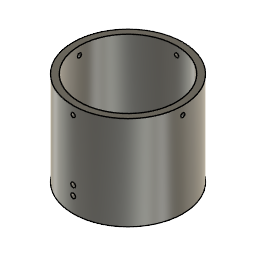
container0306v0.3 (Autodesk Fusion 360 design; units mm, degrees)
Autodesk Fusion 360 part; units mm, degrees
sketch "Sketch1" plane through (0, 0, 0) normal (0, 0, 1) x (1, 0, 0)
  circle A0 centre (0, 0) radius 31.1
  circle A1 centre (0, 0) radius 33.6
  circle A2 centre (0, 0) radius 4
  dimension "d1" = 62.2
  dimension "d2" = 67.2
  dimension "d16" = 8
  constraint coincident A0.centre A1.centre
  constraint concentric A0 A1
  measures "d1" diameter of A0
  measures "d2" diameter of A1
  measures "d16" diameter of A2
extrude "Extrude1" add sketch "Sketch1" along normal blind 60 contours A1
extrude "Extrude2" add sketch "Sketch1" along normal blind 4 contours A0 | A2
ref_plane "WorkPlane1" through (0, -35, 0) normal (0, 1, 0) x (0, 0, 1)
sketch "Sketch2" plane through (0, -35, 0) normal (0, 1, 0) x (1, 0, 0)
  circle A0 centre (0, -10) radius 1.5
  circle A1 centre (0, -16) radius 1.5
  circle A2 centre (0, -54.7) radius 1.3
  line L0 (0, 0) -> (0, -53.4)
  dimension "d25" = 3
  dimension "d26" = 6
  dimension "d27" = 3
  dimension "d32" = 2.6
  constraint coincident L0.start origin
  constraint vertical L0
  constraint coincident A2 L0.end
  measures "d25" diameter of A0
  measures "d26" distance of A0.centre A1.centre
  measures "d27" diameter of A1
  measures "d32" diameter of A2
hole "Hole2" at (0, 0, 0) direction (0, 0, 1) diameter 8 depth 8 tip angle 118
extrude "Extrude4" cut sketch "Sketch2" along normal blind 85 contours A0 L0 | A0 L0 | A1 L0 | A1 L0
extrude "Extrude5" cut sketch "Sketch2" along normal blind 14 contours A2
pattern_circular "C-Pattern2" count 4 over 360 about axis through (0, 0, 1.75) along (0, 0, 1) of 1 faces at (0.3204, -31.9316, 53.4401)
move_face "OffsetFaces1" offset 1.5 1 faces at (5.4983, 33.1471, 25.3921)
